Thermoformable caliper hanging bracket (Autodesk Fusion 360 design; units mm, degrees)
Autodesk Fusion 360 part; units mm, degrees
sketch "Sketch1" plane through (0, 0, 0) normal (0, 0, 1) x (1, 0, 0)
  line L0 (56, 13.5) -> (56, 28)
  line L1 (56, 28) -> (0, 28)
  line L2 (0, 28) -> (0, 0)
  line L3 (0, 0) -> (10, 0)
  line L4 (10, 0) -> (46, 0) construction
  line L5 (0, 0) -> (0, -35)
  arc A0 (0, -35) -> (10, -35) centre (5, -35) ccw
  line L6 (10, -35) -> (10, 0)
  line L7 (46, 0) -> (46, 13.5) construction
  line L8 (46, 13.5) -> (56, 13.5)
  line L9 (46, 13.5) -> (10, 0)
  line L10 (46, 13.5) -> (46, -21.5)
  arc A1 (46, -21.5) -> (56, -21.5) centre (51, -21.5) ccw
  line L11 (56, -21.5) -> (56, 13.5)
  line L12 (0, -33) -> (10, -33) construction
  line L13 (46, -19.5) -> (56, -19.5) construction
  line L14 (46, 15.5) -> (56, 15.5)
  line L15 (0, 2) -> (10, 2)
  line L16 (0, -32) -> (10, -32)
  line L17 (0, -34) -> (10, -34)
  line L18 (46, -18.5) -> (56, -18.5)
  line L19 (46, -20.5) -> (56, -20.5)
  line L20 (46, 15.5) -> (46, 13.5)
  line L21 (46, 15.5) -> (45.6, 15.5)
  line L22 (45.6, 15.5) -> (45.6, 13.35)
  line L23 (10, 0) -> (10, 2)
  line L24 (10, 2) -> (10.4, 2)
  line L25 (10.4, 2) -> (10.4, 0.15)
  dimension "d1" = 28
  dimension "d5" = 10
  dimension "d6" = 10
  dimension "d7" = 36
  dimension "d8" = 13.5
  dimension "d11" = 33
  dimension "d12" = 2
  dimension "d13" = 2
  dimension "d14" = 33
  dimension "d20" = 2
  dimension "d21" = 2
  dimension "d27" = 2
  dimension "d28" = 0.4
  dimension "d29" = 2
  dimension "d30" = 0.4
  constraint horizontal L3
  constraint vertical L0
  constraint horizontal L1
  constraint vertical L2
  constraint coincident L2.end L3.start
  constraint coincident L4.end L3
  constraint perpendicular L3 L5
  constraint tangent L5 A0
  constraint vertical L6
  constraint tangent A0 L6
  constraint perpendicular L4 L7
  constraint perpendicular L0 L8
  constraint perpendicular L8 L10
  constraint tangent L10 A1
  constraint vertical L11
  constraint tangent A1 L11
  constraint coincident L5 L12.start
  constraint coincident L6 L12.end
  constraint perpendicular L6 L12
  constraint coincident L10 L13.start
  constraint coincident L11 L13.end
  constraint perpendicular L11 L13
  constraint coincident L10 L14.start
  constraint coincident L11 L14.end
  constraint perpendicular L11 L14
  constraint coincident L5 L15.start
  constraint coincident L6 L15.end
  constraint perpendicular L6 L15
  constraint coincident L5 L16.start
  constraint coincident L6 L16.end
  constraint perpendicular L6 L16
  constraint coincident L5 L17.start
  constraint coincident L6 L17.end
  constraint perpendicular L6 L17
  constraint symmetric L12 L16 L17
  constraint coincident L10 L18.start
  constraint coincident L11 L18.end
  constraint perpendicular L11 L18
  constraint coincident L10 L19.start
  constraint coincident L11 L19.end
  constraint perpendicular L11 L19
  constraint symmetric L13 L18 L19
  constraint perpendicular L20 L21
  constraint coincident L9 L22.end
  constraint perpendicular L21 L22
  constraint perpendicular L23 L24
  constraint coincident L9 L25.end
  constraint perpendicular L24 L25
  measures "d1" distance of L2.end L1.end
  measures "d5" distance of L2.end L3.end
  measures "d6" distance of L0 L4.end
  measures "d7" distance of L3.end L4.end
  measures "d8" distance of L4.end L7.end
  measures "d11" distance of L2.end L12.start
  measures "d12" distance of L5.end L12.start
  measures "d13" distance of L10.end L13.start
  measures "d14" distance of L7.end L13.start
  measures "d20" distance of L16 L17
  measures "d21" distance of L18 L19
  measures "d27" distance of L3 L15
  measures "d28" distance of L14.start L21.end
  measures "d29" distance of L8 L14
  measures "d30" distance of L15.end L24.end
extrude "Extrude1" add sketch "Sketch1" against normal blind 3 contours L0 L8 L14 L20 | L8 L10 L11 L18 | L0 L1 L2 L9 L14 L15 L21 L22 L24 L25 | L10 L11 L18 L19 | L10 A1 L11 L19 | L2 L3 L15 L23 | L3 L5 L6 L16 | L5 L6 L16 L17 | L5 A0 L6 L17
extrude "Extrude2" cut sketch "Sketch1" against normal blind 1 contours L0 L8 L14 L20 | L10 L11 L18 L19 | L2 L3 L15 L23 | L5 L6 L16 L17
chamfer "Chamfer1" distance 1 angle 45 8 edges at (5, -32, -1) (5, -34, -1) (5, 2, -1) (5, 0, -1) (51, 13.5, -1) (51, 15.5, -1) (51, -20.5, -1) (51, -18.5, -1)
fillet "Fillet1" radius 5 2 edges at (56, 28, -1.5) (0, 28, -1.5)
equation "d13 = d12"
equation "d14 = d11"
